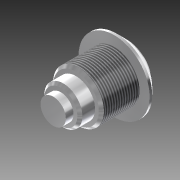
# Autodesk Inventor part: Lock
Saved by Autodesk Inventor 2015 (Build 190159000, 159)
## iProperties
Created: 2013-05-04
Part Number: Lock
Document SubType Name: Modeling
Designer: Estacion4
Density: 1 g/cm^3
Mass: 8.33901 g
Surface Area: 27.6235 cm^2
Volume: 8.33901 cm^3
Material: Generic
Appearance: Chrome - Polished
Author: Estacion4
Autodesk Inventor part; units mm, degrees
ref_plane "YZ Plane" through (0, 0, 0) normal (1, 0, 0) x (0, 1, 0)
ref_plane "XZ Plane" through (0, 0, 0) normal (0, 1, 0) x (-1, 0, 0)
ref_plane "XY Plane" through (0, 0, 0) normal (0, 0, 1) x (1, 0, 0)
sketch "Boceto1" plane through (0, 0, 0) normal (0, 0, 1) x (1, 0, 0)
  line L0 (0, 0) -> (0, -28)
  line L1 (0, 0) -> (-11, 0)
  line L2 (-11, 0) -> (-14, -3)
  line L3 (-14, -3) -> (-14, -4)
  line L4 (-14, -4) -> (-10, -4)
  line L5 (-10, -4) -> (-10, -19)
  line L6 (-10, -19) -> (-7.5, -19)
  line L7 (-7.5, -19) -> (-7.5, -25)
  line L8 (-7.5, -25) -> (-5, -25)
  line L9 (-5, -25) -> (-5, -28)
  line L10 (-5, -28) -> (0, -28)
  dimension "d0" = 28
  dimension "d1" = 45
  dimension "d2" = 4
  dimension "d3" = 1
  dimension "d5" = 28
  dimension "d6" = 20
  dimension "d7" = 15
  dimension "d8" = 10
  dimension "d9" = 15
  dimension "d10" = 6
  constraints: 22 end point, 5 parallel, 4 perpendicular, 1 vertical
  measures "d0" diameter of L3 L0
  measures "d1" angle of L1 L2
  measures "d2" distance between parallel lines of L4 L1
  measures "d3" distance of L2.end L3.end
  measures "d5" distance of L0.start L0.end
  measures "d6" diameter of L5 L0
  measures "d7" diameter of L7 L0
  measures "d8" diameter of L9 L0
  measures "d9" distance between parallel lines of L6 L4
  measures "d10" distance of L6.end L7.end
revolve "Revolución1" add sketch "Boceto1" angle 360 about axis through (0, 0, 0) along (0, -1, 0)
thread "Rosca1" size "M20x1" class "6g" standard "ANSI Metric M Profile" full length
chamfer "Chaflán1" distance 1 angle 45 2 edges at (10, -19, 0) (7.5, -25, 0)
sketch "Boceto2" plane through (0, 0, 0) normal (0, 1, 0) x (1, 0, 0)
  circle A0 centre (0, 0) radius 11 projected
  circle A1 centre (0, 0) radius 10
  dimension "d17" = 1
  constraints: 1 centre point, 1 coincident
  measures "d17" radial gap between concentric circles of A0 A1
extrude "Extrusión1" add sketch "Boceto2" along normal blind 1 contours A1
sketch "Boceto3" plane through (0, 1, 0) normal (0, 1, 0) x (1, 0, 0)
  circle A0 centre (0, 0) radius 10 projected
  line L0 (6.5, 1) -> (-6.5, 1)
  line L1 (-6.5, 1) -> (-6.5, -1)
  line L2 (-6.5, -1) -> (6.5, -1)
  line L3 (6.5, -1) -> (6.5, 1)
  point P0 (0, 1)
  point P1 (6.5, 0)
  dimension "d20" = 2
  dimension "d21" = 13
  constraints: 8 end point, 2 midpoint, 2 parallel, 1 horizontal, 1 horizontal alignment, 1 perpendicular, 1 vertical alignment
  measures "d20" distance of L0.end L1.end
  measures "d21" distance of L1.end L2.end
extrude "Extrusión2" cut sketch "Boceto3" against normal blind 1 contours L3 L2 L1 L0
body "Solid1"
